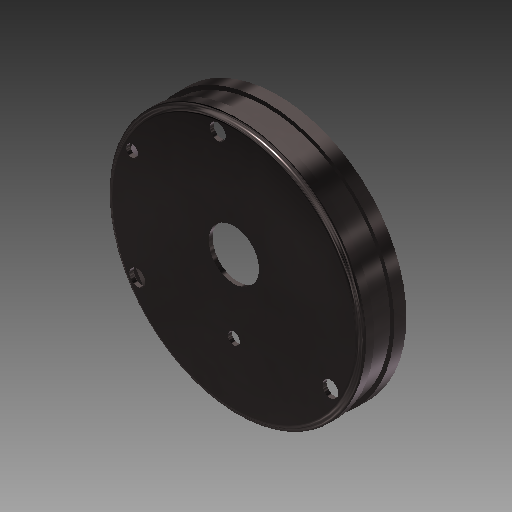
# Autodesk Inventor part: 407-02
Saved by Autodesk Inventor 2019 (Build 230136000, 136)
## iProperties
Company: Autodesk Inc.
Created: 2017-06-27
Part Number: 407-02
Material: Stainless Steel
Document SubType Name: Modeling
Designer: Autodesk Inc.
Density: 8 g/cm^3
Appearance: Anodized - Subtle Dark Bronze
Mass: 41.7849 g
Surface Area: 107.538 cm^2
Volume: 5.22311 cm^3
Author: Inventor
Autodesk Inventor part; units mm, degrees
ref_plane "YZ Plane" through (0, 0, 0) normal (1, 0, 0) x (0, 1, 0)
ref_plane "XZ Plane" through (0, 0, 0) normal (0, 1, 0) x (-1, 0, 0)
ref_plane "XY Plane" through (0, 0, 0) normal (0, 0, 1) x (1, 0, 0)
sketch "Sketch1" plane through (0, 0, 0) normal (0, 0, 1) x (1, 0, 0)
  circle A0 centre (0, 0) radius 31.875
  dimension "d0" = 63.75
  constraints: 1 centre point, 1 coincident
  measures "d0" diameter of A0
extrude "Extrusion1" add sketch "Sketch1" along normal blind 11
sketch "Sketch6" plane through (0, 0, 0) normal (1, 0, 0) x (0, 1, 0)
  line L0 (30.875, 8) -> (31.875, 8)
  line L1 (31.875, 8) -> (31.875, 3)
  line L2 (31.875, 3) -> (30.875, 3)
  line L3 (30.875, 3) -> (30.875, 8)
  line L4 (0, 0) -> (0, 11) construction
  line L5 (31.875, 11) -> (-31.875, 11) projected
  line L6 (-31.875, 0) -> (31.875, 0) projected
  circle A0 centre (31.875, 11) radius 1
  dimension "d62" = 1
  dimension "d63" = 5
  dimension "d65" = 31.875
  dimension "d66" = 63.75
  dimension "d67" = 3
  dimension "d81" = 2
  constraints: 10 end point, 2 parallel, 1 centre point, 1 coincident, 1 horizontal, 1 midpoint, 1 perpendicular
  measures "d62" distance of L1.end L2.end
  measures "d63" distance of L0.end L1.end
  measures "d65" distance from line of L4 L1.end
  measures "d66" distance of L5.start L5.end
  measures "d67" distance between parallel lines of L6 L2
  measures "d81" diameter of A0
revolve "Revolution1" cut sketch "Sketch6" angle 360 about axis through (0, 0, 0) along (0, 0, 1)
shell "Shell1" thickness 1 removed faces 1 at (5.5896, -2.5427, 0)
sketch "Sketch2" plane through (0, 0, 11) normal (0, 0, 1) x (1, 0, 0)
  circle A0 centre (0, 0) radius 31.875 projected
  point P0 (-4, 27.5)
  point P1 (-24, -13.9)
  point P2 (24, -13.9)
  dimension "d73" = 4
  dimension "d74" = 27.5
  dimension "d77" = 13.9
  dimension "d78" = 24
  dimension "d79" = 13.9
  dimension "d80" = 24
  measures "d73" horizontal distance of A0.centre point (-4, 27.5)
  measures "d74" vertical distance of A0.centre point (-4, 27.5)
  measures "d77" vertical distance of point (-24, -13.9) A0.centre
  measures "d78" horizontal distance of A0.centre point (-24, -13.9)
  measures "d79" vertical distance of point (24, -13.9) A0.centre
  measures "d80" horizontal distance of point (24, -13.9) A0.centre
hole "Hole1" at (-4, 27.5, 11) at (24, -13.9, 11) at (-24, -13.9, 11) direction (0, 0, -1) diameter 4 end through all
sketch "Sketch3" plane through (0, 0, 11) normal (0, 0, 1) x (1, 0, 0)
  circle A0 centre (0, 0) radius 31.875 projected
  point P0 (-25.3, 12.7)
  dimension "d31" = 25.3
  dimension "d32" = 12.7
  measures "d31" horizontal distance of point (-25.3, 12.7) A0.centre
  measures "d32" vertical distance of point (-25.3, 12.7) A0.centre
hole "Hole2" at (-25.3, 12.7, 11) direction (0, 0, -1) diameter 3 end through all
sketch "Sketch4" plane through (0, 0, 11) normal (0, 0, 1) x (1, 0, 0)
  point P0 (0, 0)
  point P1 (0, 3)
  dimension "d40" = 3
  constraints: 1 vertical alignment
  measures "d40" distance of point (0, 3) point (0, 0)
hole "Hole3" at (0, 3, 11) direction (0, 0, -1) diameter 12.5 end through all
sketch "Sketch5" plane through (0, 0, 11) normal (0, 0, 1) x (1, 0, 0)
  point P0 (0, 0)
  point P1 (0, -15)
  dimension "d48" = 15
  constraints: 1 vertical alignment
  measures "d48" distance of point (0, 0) point (0, -15)
hole "Hole4" at (0, -15, 11) direction (0, 0, -1) diameter 3 end through all
fillet "Fillet1" radius 1 1 edges at (0, -30.875, 11)
sketch "Sketch7" plane through (0, 0, 0) normal (0, 0, -1) x (-1, 0, 0)
  line L0 (0, 0) -> (28, 0) construction
  line L1 (28, -5) -> (28, 5) construction
  circle A0 centre (28, -5) radius 2.5
  circle A1 centre (28, 5) radius 2.5
  circle A2 centre (0, 0) radius 31.009 projected
  dimension "d83" = 28
  dimension "d84" = 10
  dimension "d85" = 5
  dimension "d86" = 5
  constraints: 4 end point, 2 centre point, 2 coincident, 1 horizontal, 1 midpoint, 1 vertical
  measures "d83" distance of L0.end L0.start
  measures "d84" distance of L1.start L1.end
  measures "d85" diameter of A0
  measures "d86" diameter of A1
extrude "Extrusion2" cut sketch "Sketch7" against normal blind 2 contours A0 | A1
fillet "Fillet2" radius 2 2 edges at (-30.4611, -5.4395, 0) (-30.4611, 5.4395, 0)
equation "\"d65\" = 0.5 * d66"
equation "\"d77\" = d79"
equation "\"d78\" = d80"
body "Solid1"
